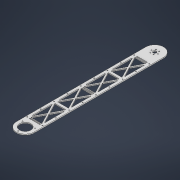
# Autodesk Inventor part: Lower_Arm_Motor_Side
Saved by Autodesk Inventor 2022 (Build 260153000, 153)
## iProperties
Created: 2023-02-15
Part Number: Lower_Arm_Motor_Side
Material: Generic
Document SubType Name: Modeling
Designer: dzw04
Density: 1 g/cm^3
Appearance: Default
Author: dzw04
Autodesk Inventor part; units mm, degrees
ref_plane "YZ Plane" through (0, 0, 0) normal (1, 0, 0) x (0, 1, 0)
ref_plane "XZ Plane" through (0, 0, 0) normal (0, 1, 0) x (-1, 0, 0)
ref_plane "XY Plane" through (0, 0, 0) normal (0, 0, 1) x (1, 0, 0)
sketch "Sketch1" plane through (0, 0, 0) normal (0, 1, 0) x (-1, 0, 0)
  line L0 (27.5, 400) -> (27.5, 0)
  arc A0 (-27.5, 0) -> (27.5, 0) centre (0, 0) ccw
  line L1 (-27.5, 0) -> (-27.5, 400)
  arc A1 (27.5, 400) -> (-27.5, 400) centre (0, 400) ccw
  circle A2 centre (23.5, 370) radius 1.5
  circle A3 centre (-23.25, 370) radius 1.5
  circle A4 centre (0, 400) radius 17.5
  circle A5 centre (0, 422) radius 1.5
  circle A6 centre (19.0526, 389) radius 1.5
  circle A7 centre (-19.0526, 389) radius 1.5
  circle A8 centre (23.5, 246.25) radius 1.5
  arc A9 (-2.5003, 328.2862) -> (-2.5003, 329.2138) centre (-3.3862, 328.75) ccw
  line L2 (-2.5003, 329.2138) -> (-17.6141, 358.085)
  arc A10 (-17.6141, 358.085) -> (-19.5, 357.6212) centre (-18.5, 357.6212) ccw
  line L3 (-19.5, 357.6212) -> (-19.5, 299.8788)
  arc A11 (-19.5, 299.8788) -> (-17.6141, 299.415) centre (-18.5, 299.8788) ccw
  line L4 (-17.6141, 299.415) -> (-2.5003, 328.2862)
  circle A12 centre (-23.25, 328.75) radius 1.5
  line L5 (-17.6141, 134.415) -> (-2.5003, 163.2862)
  arc A13 (-2.5003, 163.2862) -> (-2.5003, 164.2138) centre (-3.3862, 163.75) ccw
  line L6 (-2.5003, 164.2138) -> (-17.6141, 193.085)
  arc A14 (-17.6141, 193.085) -> (-19.5, 192.6212) centre (-18.5, 192.6212) ccw
  line L7 (-19.5, 192.6212) -> (-19.5, 134.8788)
  arc A15 (-19.5, 134.8788) -> (-17.6141, 134.415) centre (-18.5, 134.8788) ccw
  circle A16 centre (23.5, 81.25) radius 1.5
  circle A17 centre (-23.25, 122.5) radius 1.5
  arc A18 (15.5903, 44) -> (16.4763, 45.4638) centre (15.5903, 45) ccw
  line L8 (16.4763, 45.4638) -> (0.8859, 75.2453)
  arc A19 (0.8859, 75.2453) -> (-0.8859, 75.2453) centre (0, 74.7815) ccw
  line L9 (-0.8859, 75.2453) -> (-16.4763, 45.4638)
  arc A20 (-16.4763, 45.4638) -> (-15.5903, 44) centre (-15.5903, 45) ccw
  line L10 (-15.5903, 44) -> (15.5903, 44)
  arc A21 (17.6141, 299.415) -> (19.5, 299.8788) centre (18.5, 299.8788) ccw
  line L11 (19.5, 299.8788) -> (19.5, 357.6212)
  arc A22 (19.5, 357.6212) -> (17.6141, 358.085) centre (18.5, 357.6212) ccw
  line L12 (17.6141, 358.085) -> (2.5003, 329.2138)
  arc A23 (2.5003, 329.2138) -> (2.5003, 328.2862) centre (3.3862, 328.75) ccw
  line L13 (2.5003, 328.2862) -> (17.6141, 299.415)
  line L14 (-2.5003, 246.7138) -> (-17.6141, 275.585)
  arc A24 (-17.6141, 275.585) -> (-19.5, 275.1212) centre (-18.5, 275.1212) ccw
  line L15 (-19.5, 275.1212) -> (-19.5, 217.3788)
  arc A25 (-19.5, 217.3788) -> (-17.6141, 216.915) centre (-18.5, 217.3788) ccw
  line L16 (-17.6141, 216.915) -> (-2.5003, 245.7862)
  arc A26 (-2.5003, 245.7862) -> (-2.5003, 246.7138) centre (-3.3862, 246.25) ccw
  arc A27 (16.4763, 282.0362) -> (15.5903, 283.5) centre (15.5903, 282.5) ccw
  line L17 (15.5903, 283.5) -> (-15.5903, 283.5)
  arc A28 (-15.5903, 283.5) -> (-16.4763, 282.0362) centre (-15.5903, 282.5) ccw
  line L18 (-16.4763, 282.0362) -> (-0.8859, 252.2547)
  arc A29 (-0.8859, 252.2547) -> (0.8859, 252.2547) centre (0, 252.7185) ccw
  line L19 (0.8859, 252.2547) -> (16.4763, 282.0362)
  arc A30 (-0.8859, 169.7547) -> (0.8859, 169.7547) centre (0, 170.2185) ccw
  line L20 (0.8859, 169.7547) -> (16.4763, 199.5362)
  arc A31 (16.4763, 199.5362) -> (15.5903, 201) centre (15.5903, 200) ccw
  line L21 (15.5903, 201) -> (-15.5903, 201)
  arc A32 (-15.5903, 201) -> (-16.4763, 199.5362) centre (-15.5903, 200) ccw
  line L22 (-16.4763, 199.5362) -> (-0.8859, 169.7547)
  line L23 (-16.4763, 117.0362) -> (-0.8859, 87.2547)
  arc A33 (-0.8859, 87.2547) -> (0.8859, 87.2547) centre (0, 87.7185) ccw
  line L24 (0.8859, 87.2547) -> (16.4763, 117.0362)
  arc A34 (16.4763, 117.0362) -> (15.5903, 118.5) centre (15.5903, 117.5) ccw
  line L25 (15.5903, 118.5) -> (-15.5903, 118.5)
  arc A35 (-15.5903, 118.5) -> (-16.4763, 117.0362) centre (-15.5903, 117.5) ccw
  circle A36 centre (-23.25, 246.25) radius 1.5
  line L26 (17.6141, 193.085) -> (2.5003, 164.2138)
  arc A37 (2.5003, 164.2138) -> (2.5003, 163.2862) centre (3.3862, 163.75) ccw
  line L27 (2.5003, 163.2862) -> (17.6141, 134.415)
  arc A38 (17.6141, 134.415) -> (19.5, 134.8788) centre (18.5, 134.8788) ccw
  line L28 (19.5, 134.8788) -> (19.5, 192.6212)
  arc A39 (19.5, 192.6212) -> (17.6141, 193.085) centre (18.5, 192.6212) ccw
  circle A40 centre (23.5, 287.5) radius 1.5
  circle A41 centre (-23.25, 163.75) radius 1.5
  circle A42 centre (-23.25, 81.25) radius 1.5
  line L29 (-2.5003, 81.7138) -> (-17.6141, 110.585)
  arc A43 (-17.6141, 110.585) -> (-19.5, 110.1212) centre (-18.5, 110.1212) ccw
  line L30 (-19.5, 110.1212) -> (-19.5, 52.3788)
  arc A44 (-19.5, 52.3788) -> (-17.6141, 51.915) centre (-18.5, 52.3788) ccw
  line L31 (-17.6141, 51.915) -> (-2.5003, 80.7862)
  arc A45 (-2.5003, 80.7862) -> (-2.5003, 81.7138) centre (-3.3862, 81.25) ccw
  line L32 (2.5003, 80.7862) -> (17.6141, 51.915)
  arc A46 (17.6141, 51.915) -> (19.5, 52.3788) centre (18.5, 52.3788) ccw
  line L33 (19.5, 52.3788) -> (19.5, 110.1212)
  arc A47 (19.5, 110.1212) -> (17.6141, 110.585) centre (18.5, 110.1212) ccw
  line L34 (17.6141, 110.585) -> (2.5003, 81.7138)
  arc A48 (2.5003, 81.7138) -> (2.5003, 80.7862) centre (3.3862, 81.25) ccw
  line L35 (0.8859, 334.7547) -> (16.4763, 364.5362)
  arc A49 (16.4763, 364.5362) -> (15.5903, 366) centre (15.5903, 365) ccw
  line L36 (15.5903, 366) -> (-15.5903, 366)
  arc A50 (-15.5903, 366) -> (-16.4763, 364.5362) centre (-15.5903, 365) ccw
  line L37 (-16.4763, 364.5362) -> (-0.8859, 334.7547)
  arc A51 (-0.8859, 334.7547) -> (0.8859, 334.7547) centre (0, 335.2185) ccw
  circle A52 centre (23.5, 205) radius 1.5
  arc A53 (0.8859, 157.7453) -> (-0.8859, 157.7453) centre (0, 157.2815) ccw
  line L38 (-0.8859, 157.7453) -> (-16.4763, 127.9638)
  arc A54 (-16.4763, 127.9638) -> (-15.5903, 126.5) centre (-15.5903, 127.5) ccw
  line L39 (-15.5903, 126.5) -> (15.5903, 126.5)
  arc A55 (15.5903, 126.5) -> (16.4763, 127.9638) centre (15.5903, 127.5) ccw
  line L40 (16.4763, 127.9638) -> (0.8859, 157.7453)
  line L41 (-15.5903, 291.5) -> (15.5903, 291.5)
  arc A56 (15.5903, 291.5) -> (16.4763, 292.9638) centre (15.5903, 292.5) ccw
  line L42 (16.4763, 292.9638) -> (0.8859, 322.7453)
  arc A57 (0.8859, 322.7453) -> (-0.8859, 322.7453) centre (0, 322.2815) ccw
  line L43 (-0.8859, 322.7453) -> (-16.4763, 292.9638)
  arc A58 (-16.4763, 292.9638) -> (-15.5903, 291.5) centre (-15.5903, 292.5) ccw
  circle A59 centre (23.5, 122.5) radius 1.5
  circle A60 centre (-23.25, 205) radius 1.5
  arc A61 (15.5903, 209) -> (16.4763, 210.4638) centre (15.5903, 210) ccw
  line L44 (16.4763, 210.4638) -> (0.8859, 240.2453)
  arc A62 (0.8859, 240.2453) -> (-0.8859, 240.2453) centre (0, 239.7815) ccw
  line L45 (-0.8859, 240.2453) -> (-16.4763, 210.4638)
  arc A63 (-16.4763, 210.4638) -> (-15.5903, 209) centre (-15.5903, 210) ccw
  line L46 (-15.5903, 209) -> (15.5903, 209)
  circle A64 centre (23.5, 163.75) radius 1.5
  arc A65 (-15, 206.5) -> (-15, 203.5) centre (-15, 205) ccw
  line L47 (-15, 203.5) -> (15, 203.5)
  arc A66 (15, 203.5) -> (15, 206.5) centre (15, 205) ccw
  line L48 (15, 206.5) -> (-15, 206.5)
  circle A67 centre (23.5, 328.75) radius 1.5
  circle A68 centre (-23.25, 287.5) radius 1.5
  arc A69 (19.5, 275.1212) -> (17.6141, 275.585) centre (18.5, 275.1212) ccw
  line L49 (17.6141, 275.585) -> (2.5003, 246.7138)
  arc A70 (2.5003, 246.7138) -> (2.5003, 245.7862) centre (3.3862, 246.25) ccw
  line L50 (2.5003, 245.7862) -> (17.6141, 216.915)
  arc A71 (17.6141, 216.915) -> (19.5, 217.3788) centre (18.5, 217.3788) ccw
  line L51 (19.5, 217.3788) -> (19.5, 275.1212)
  circle A72 centre (23.5, 40) radius 1.5
  line L52 (-15, 38.5) -> (15, 38.5)
  arc A73 (15, 38.5) -> (15, 41.5) centre (15, 40) ccw
  line L53 (15, 41.5) -> (-15, 41.5)
  arc A74 (-15, 41.5) -> (-15, 38.5) centre (-15, 40) ccw
  circle A75 centre (-23.25, 40) radius 1.5
  line L54 (15, 371.5) -> (-15, 371.5)
  arc A76 (-15, 371.5) -> (-15, 368.5) centre (-15, 370) ccw
  line L55 (-15, 368.5) -> (15, 368.5)
  arc A77 (15, 368.5) -> (15, 371.5) centre (15, 370) ccw
  circle A78 centre (-5, 8.6603) radius 1.5
  circle A79 centre (-10, 0) radius 1.5
  circle A80 centre (5, 8.6603) radius 1.5
  circle A81 centre (-5, -8.6603) radius 1.5
  circle A82 centre (10, 0) radius 1.5
  circle A83 centre (5, -8.6603) radius 1.5
  circle A84 centre (0, 0) radius 5
  point P0 (15, 368.5)
  point P1 (-15, 368.5)
  point P2 (-15, 371.5)
  point P3 (2.5003, 245.7862)
  point P4 (17.6141, 275.585)
  point P5 (15, 206.5)
  point P6 (15, 203.5)
  point P7 (-15.5903, 209)
  point P8 (-0.8859, 240.2453)
  point P9 (16.4763, 210.4638)
  point P10 (-0.8859, 322.7453)
  point P11 (0.8859, 322.7453)
  point P12 (16.4763, 292.9638)
  point P13 (15.5903, 291.5)
  point P14 (0.8859, 157.7453)
  point P15 (-0.8859, 157.7453)
  point P16 (-16.4763, 364.5362)
  point P17 (19.5, 52.3788)
  point P18 (-2.5003, 80.7862)
  point P19 (-17.6141, 51.915)
  point P20 (2.5003, 163.2862)
  point P21 (15.5903, 118.5)
  point P22 (0.8859, 87.2547)
  point P23 (-0.8859, 169.7547)
  point P24 (-16.4763, 199.5362)
  point P25 (0.8859, 169.7547)
  point P26 (0.8859, 252.2547)
  point P27 (-16.4763, 282.0362)
  point P28 (-15.5903, 283.5)
  point P29 (-2.5003, 245.7862)
  point P30 (-17.6141, 216.915)
  point P31 (17.6141, 299.415)
  point P32 (2.5003, 329.2138)
  point P33 (17.6141, 358.085)
  point P34 (19.5, 299.8788)
  point P35 (-0.8859, 75.2453)
  point P36 (16.4763, 45.4638)
  point P37 (-2.5003, 164.2138)
  constraints: 112 end point, 112 point on circle, 85 centre point
extrude "Extrusion1" add sketch "Sketch1" along normal blind 3
body "Solid1"
